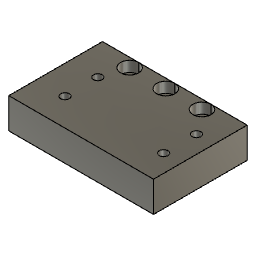
Main_Plate (Autodesk Fusion 360 design; units mm, degrees)
Autodesk Fusion 360 part; units mm, degrees
sketch "Sketch1" plane through (0, 0, 0) normal (0, 0, 1) x (1, 0, 0)
  line L0 (0, 0) -> (55.88, 0)
  line L1 (55.88, 0) -> (55.88, 36.1823)
  line L2 (0, 34.925) -> (0, 0)
  line L3 (0, 0) -> (11.0236, 0)
  line L4 (11.0236, 0) -> (11.0236, 10.668) construction
  circle A0 centre (11.0236, 10.668) radius 1.6637
  line L5 (11.0236, 10.668) -> (11.0236, 23.368) construction
  circle A1 centre (11.0236, 23.368) radius 1.6637
  line L6 (11.0236, 10.668) -> (49.1236, 10.668) construction
  line L7 (11.0236, 23.368) -> (49.1236, 23.368) construction
  circle A2 centre (49.1236, 10.668) radius 1.6637
  circle A3 centre (49.1236, 23.368) radius 1.6637
  line L8 (0, 34.925) -> (0, 30.4546)
  line L9 (0, 30.4546) -> (55.88, 30.4546) construction
  line L10 (27.94, 34.925) -> (27.94, 30.4546) construction
  line L11 (27.94, 32.6898) -> (55.88, 32.6898) construction
  line L12 (27.94, 32.6898) -> (0, 32.6898) construction
  line L13 (13.97, 32.6898) -> (13.97, 30.4546) construction
  line L14 (41.91, 32.6898) -> (41.91, 30.4546) construction
  circle A4 centre (13.97, 32.6898) radius 1.9812
  circle A5 centre (27.94, 32.6898) radius 1.9812
  circle A6 centre (41.91, 32.6898) radius 1.9812
  circle A7 centre (13.97, 32.6898) radius 3.4925
  circle A8 centre (27.94, 32.6898) radius 3.4925
  circle A9 centre (41.91, 32.6898) radius 3.4925
  line L15 (13.97, 36.1823) -> (0, 36.1823)
  line L16 (0, 36.1823) -> (0, 34.925)
  line L17 (13.97, 36.1823) -> (55.88, 36.1823)
  line L18 (0, 34.925) -> (55.88, 34.925)
  dimension "d1" = 55.88
  dimension "d2" = 34.925
  dimension "d3" = 11.0236
  dimension "d4" = 10.668
  dimension "d5" = 3.3274
  dimension "d6" = 12.7
  dimension "d7" = 3.3274
  dimension "d8" = 38.1
  dimension "d9" = 38.1
  dimension "d10" = 3.3274
  dimension "d11" = 3.3274
  dimension "d12" = 4.4704
  dimension "d13" = 3.9624
  dimension "d14" = 3.9624
  dimension "d15" = 3.9624
  dimension "d16" = 6.985
  dimension "d17" = 6.985
  dimension "d18" = 6.985
  constraint horizontal L0
  constraint vertical L1
  constraint vertical L2
  constraint coincident L0.start L2.end
  constraint perpendicular L2 L3
  constraint vertical L4
  constraint coincident L4.end A0.centre
  constraint parallel L4 L5
  constraint coincident L5.end A1.centre
  constraint perpendicular L5 L6
  constraint perpendicular L5 L7
  constraint coincident L6.end A2.centre
  constraint coincident L7.end A3.centre
  constraint coincident L1 L9.end
  constraint perpendicular L1 L9
  constraint midpoint L9 L10.end
  constraint midpoint L10 L11.start
  constraint coincident L1 L11.end
  constraint perpendicular L1 L11
  constraint midpoint L8 L12.end
  constraint midpoint L12 L13.start
  constraint coincident L9 L13.end
  constraint perpendicular L9 L13
  constraint midpoint L11 L14.start
  constraint coincident L9 L14.end
  constraint perpendicular L9 L14
  constraint coincident L13.start A4.centre
  constraint coincident L11.start L12.start
  constraint coincident L14.start A6.centre
  constraint concentric A4 A7
  constraint concentric A5 A8
  constraint concentric A6 A9
  constraint coincident A7 L15.start
  constraint tangent A7 L15
  constraint tangent A7 L17
  constraint coincident L1 L18.end
  constraint perpendicular L1 L18
  measures "d1" distance of L0.start L0.end
  measures "d2" distance of L0.start L2.start
  measures "d3" distance of L0.start L3.end
  measures "d4" distance of L3.end L4.end
  measures "d5" diameter of A0
  measures "d6" distance of L4.end L5.end
  measures "d7" diameter of A1
  measures "d8" distance of L4.end L6.end
  measures "d9" distance of L5.end L7.end
  measures "d10" diameter of A2
  measures "d11" diameter of A3
  measures "d12" distance of L2.start L8.end
  measures "d13" diameter of A4
  measures "d14" diameter of A5
  measures "d15" diameter of A6
  measures "d16" diameter of A7
  measures "d17" diameter of A8
  measures "d18" diameter of A9
extrude "Extrude1" add sketch "Sketch1" against normal blind 11.7856
extrude "Extrude2" cut sketch "Sketch1" against normal blind 4.064 contours A7 L18 | A7 L18 | A9 L18 | A9 L18 | A8 L18 | A8 L18
